Support Batterie 5V (Autodesk Fusion 360 design; units mm, degrees)
Autodesk Fusion 360 part; units mm, degrees
sketch "Sketch1" plane through (0, 0, 0) normal (0, 0, 1) x (1, 0, 0)
  circle A0 centre (0, 0) radius 11.25
  line L0 (0, 0) -> (0, -12.75) construction
  line L1 (17.5, -14.25) -> (-17.5, -14.25)
  line L2 (-17.5, -14.25) -> (-17.5, -11.25)
  line L3 (-17.5, -11.25) -> (17.5, -11.25)
  line L4 (17.5, -11.25) -> (17.5, -14.25)
  line L5 (17.5, -14.25) -> (-17.5, -11.25) construction
  line L6 (-17.5, -14.25) -> (17.5, -11.25) construction
  line L7 (11.25, -11.25) -> (13.75, -11.25)
  line L8 (13.75, -11.25) -> (13.75, 29.3)
  line L9 (11.25, 30) -> (11.25, -11.25)
  line L10 (14.45, 30) -> (14.55, 30)
  line L11 (16.75, 30) -> (16.75, 30.9)
  line L12 (15.15, 32.5) -> (12.85, 32.5)
  line L13 (11.25, 30.9) -> (11.25, 30)
  line L14 (15.25, 29.3) -> (15.25, 28)
  line L15 (15.75, 27.5) -> (16.25, 27.5)
  line L16 (16.75, 28) -> (16.75, 30)
  arc A1 (14.45, 30) -> (13.75, 29.3) centre (14.45, 29.3) ccw
  arc A2 (15.25, 29.3) -> (14.55, 30) centre (14.55, 29.3) ccw
  arc A3 (15.25, 28) -> (15.75, 27.5) centre (15.75, 28) ccw
  arc A4 (16.25, 27.5) -> (16.75, 28) centre (16.25, 28) ccw
  arc A5 (16.75, 30.9) -> (15.15, 32.5) centre (15.15, 30.9) ccw
  arc A6 (12.85, 32.5) -> (11.25, 30.9) centre (12.85, 30.9) ccw
  arc A7 (-13.75, 29.3) -> (-14.45, 30) centre (-14.45, 29.3) ccw
  line L17 (-14.45, 30) -> (-14.55, 30)
  arc A8 (-14.55, 30) -> (-15.25, 29.3) centre (-14.55, 29.3) ccw
  line L18 (-15.25, 29.3) -> (-15.25, 28)
  arc A9 (-15.75, 27.5) -> (-15.25, 28) centre (-15.75, 28) ccw
  line L19 (-15.75, 27.5) -> (-16.25, 27.5)
  arc A10 (-16.75, 28) -> (-16.25, 27.5) centre (-16.25, 28) ccw
  line L20 (-16.75, 28) -> (-16.75, 30)
  line L21 (-16.75, 30) -> (-16.75, 30.9)
  arc A11 (-15.15, 32.5) -> (-16.75, 30.9) centre (-15.15, 30.9) ccw
  line L22 (-15.15, 32.5) -> (-12.85, 32.5)
  arc A12 (-11.25, 30.9) -> (-12.85, 32.5) centre (-12.85, 30.9) ccw
  line L23 (-11.25, 30.9) -> (-11.25, 30)
  line L24 (-11.25, 30) -> (-11.25, -11.25)
  line L25 (-11.25, -11.25) -> (-13.75, -11.25)
  line L26 (-13.75, -11.25) -> (-13.75, 29.3)
  point P0 (0, -12.75)
  point P1 (16.75, 32.5)
  point P2 (16.75, 27.5)
  dimension "d1" = 22.5
  dimension "d10" = 3
  dimension "d11" = 35
  dimension "d13" = 2.5
  dimension "d14" = 30
  dimension "d16" = 5.5
  dimension "d17" = 2.5
  dimension "d19" = 2.5
  dimension "d20" = 0.7
  dimension "d21" = 0.5
  dimension "d22" = 0.5
  dimension "d23" = 1.6
  dimension "d24" = 1.5
  constraint coincident A0.centre L0.start
  constraint horizontal L1
  constraint perpendicular L1 L2
  constraint parallel L1 L3
  constraint parallel L2 L4
  constraint coincident L5 P0
  constraint coincident L6 P0
  constraint coincident P0 L0.end
  constraint tangent A0 L3
  constraint vertical L0
  constraint horizontal L7
  constraint vertical L8
  constraint vertical L9
  constraint coincident L3 L7.start
  constraint tangent A0 L9
  constraint horizontal L10
  constraint vertical L11
  constraint horizontal L12
  constraint vertical L13
  constraint vertical L14
  constraint horizontal L15
  constraint vertical L16
  constraint coincident L9.start L10
  constraint tangent L8 A1
  constraint tangent L10 A1
  constraint coincident L11.start L10
  constraint tangent L10 A2
  constraint tangent L14 A2
  constraint equal A1 A2
  constraint tangent L14 A3
  constraint tangent L15 A3
  constraint coincident P2 L15
  constraint coincident P2 L16
  constraint tangent L15 A4
  constraint tangent L16 A4
  constraint coincident P1 L11
  constraint coincident P1 L12
  constraint tangent L11 A5
  constraint tangent L12 A5
  constraint tangent L12 A6
  constraint tangent L13 A6
  constraint equal A5 A6
  constraint symmetric L0 L7.start L24.end
  constraint symmetric L0 L7.end L25.end
  constraint symmetric L0 L9.start L23.end
  constraint symmetric L0 L11.start L20.end
  constraint symmetric L0 L8.end A7.start
  constraint symmetric L0 L10.start A7.end
  constraint symmetric L0 A1 A7
  constraint symmetric L0 L10.end L17.end
  constraint symmetric L0 L14.start A8.end
  constraint symmetric L0 A2 A8
  constraint symmetric L0 L14.end L18.end
  constraint symmetric L0 L15.start A9.start
  constraint symmetric L0 A3 A9
  constraint symmetric L0 L15.end L19.end
  constraint symmetric L0 L16.start A10.start
  constraint symmetric L0 A4 A10
  constraint symmetric L0 L11.end L21.end
  constraint symmetric L0 L12.start A11.start
  constraint symmetric L0 A5 A11
  constraint symmetric L0 L12.end L22.end
  constraint symmetric L0 L13.start A12.start
  constraint symmetric L0 A6 A12
  measures "d1" diameter of A0
  measures "d10" distance of L1.end L2.end
  measures "d11" distance of L1.start L1.end
  measures "d13" distance of L7.start L7.end
  measures "d14" vertical distance of A0.centre L9.start
  measures "d16" distance of L9.start L11.start
  measures "d17" distance of L11.start P1
  measures "d19" distance of L11.start P2
  measures "d20" radius of A1
  measures "d21" radius of A3
  measures "d22" radius of A4
  measures "d23" radius of A5
  measures "d24" distance of L14 L16
extrude "Extrude1" add sketch "Sketch1" along normal blind 30 contours A0 L3 L9 | L3 L7 L8 L9 L10 L11 L12 L13 L14 L15 L16 A1 A2 A3 A4 A5 A6 | L3 A7 L17 A8 L18 A9 L19 A10 L20 L21 A11 L22 A12 L23 L24 L25 L26 | A0 L3 L24 | L1 L2 L3 L4 L7 L25
fillet "Fillet1" radius 7.5 2 edges at (-13.75, -11.25, 15) (13.75, -11.25, 15)
sketch "Sketch2" plane through (0, -14.25, 0) normal (0, -1, 0) x (1, 0, 0)
  line L0 (-17.5, 0) -> (17.5, 0)
  line L1 (17.5, 0) -> (17.5, 30)
  line L2 (17.5, 30) -> (-17.5, 30)
  line L3 (-17.5, 30) -> (-17.5, 0)
  line L4 (0, 0) -> (0, 18) construction
  line L5 (-5, 18) -> (5, 18)
  circle A0 centre (-5, 18) radius 1.5
  circle A1 centre (5, 18) radius 1.5
  dimension "d29" = 18
  dimension "d30" = 10
  dimension "d31" = 3
  dimension "d32" = 3
  constraint coincident L4.start origin
  constraint perpendicular L0 L4
  constraint perpendicular L4 L5
  constraint coincident L4.end L5
  constraint midpoint L4.end L5
  constraint coincident L5.start A0.centre
  constraint coincident L5.end A1.centre
  measures "d29" distance of L4.start L4.end
  measures "d30" distance of L5.start L5.end
  measures "d31" diameter of A0
  measures "d32" diameter of A1
extrude "Extrude2" cut sketch "Sketch2" against normal through all contours A0 | A1
ref_plane "WorkPlane1" through (0, -11.25, 15) normal (0, -1, 0) x (1, 0, 0)
sketch "Sketch4" plane through (0, -11.25, 15) normal (0, -1, 0) x (1, 0, 0)
  circle A0 centre (-5, 3) radius 1.5
  circle A1 centre (5, 3) radius 1.5
  circle A2 centre (-5, 3) radius 3
  circle A3 centre (5, 3) radius 3
  dimension "d38" = 6
  dimension "d39" = 6
  constraint concentric A0 A2
  constraint concentric A1 A3
  measures "d38" diameter of A2
  measures "d39" diameter of A3
extrude "Extrude4" cut sketch "Sketch4" against normal blind 14
sketch "Sketch5" plane through (0, 0, 0) normal (0, 0, -1) x (1, 0, 0)
  arc A0 (17.5, 11.25) -> (13.75, 4.7548) centre (21.25, 4.7548) ccw
  line L0 (17.5, 11.25) -> (17.5, 14.25)
  line L1 (17.5, 14.25) -> (-17.5, 14.25)
  line L2 (-17.5, 14.25) -> (-17.5, 11.25)
  arc A1 (-13.75, 4.7548) -> (-17.5, 11.25) centre (-21.25, 4.7548) ccw
  line L3 (-13.75, 4.7548) -> (-13.75, -29.3)
  arc A2 (-14.45, -30) -> (-13.75, -29.3) centre (-14.45, -29.3) ccw
  line L4 (-14.45, -30) -> (-14.55, -30)
  arc A3 (-15.25, -29.3) -> (-14.55, -30) centre (-14.55, -29.3) ccw
  line L5 (-15.25, -29.3) -> (-15.25, -28)
  arc A4 (-15.25, -28) -> (-15.75, -27.5) centre (-15.75, -28) ccw
  line L6 (-15.75, -27.5) -> (-16.25, -27.5)
  arc A5 (-16.25, -27.5) -> (-16.75, -28) centre (-16.25, -28) ccw
  line L7 (-16.75, -28) -> (-16.75, -30.9)
  arc A6 (-16.75, -30.9) -> (-15.15, -32.5) centre (-15.15, -30.9) ccw
  line L8 (-15.15, -32.5) -> (-12.85, -32.5)
  arc A7 (-12.85, -32.5) -> (-11.25, -30.9) centre (-12.85, -30.9) ccw
  line L9 (-11.25, -30.9) -> (-11.25, 0)
  arc A8 (11.25, 0) -> (-11.25, 0) centre (0, 0) ccw
  line L10 (11.25, 0) -> (11.25, -30.9)
  arc A9 (11.25, -30.9) -> (12.85, -32.5) centre (12.85, -30.9) ccw
  line L11 (12.85, -32.5) -> (15.15, -32.5)
  arc A10 (15.15, -32.5) -> (16.75, -30.9) centre (15.15, -30.9) ccw
  line L12 (16.75, -30.9) -> (16.75, -28)
  arc A11 (16.75, -28) -> (16.25, -27.5) centre (16.25, -28) ccw
  line L13 (16.25, -27.5) -> (15.75, -27.5)
  arc A12 (15.75, -27.5) -> (15.25, -28) centre (15.75, -28) ccw
  line L14 (15.25, -28) -> (15.25, -29.3)
  arc A13 (14.55, -30) -> (15.25, -29.3) centre (14.55, -29.3) ccw
  line L15 (14.55, -30) -> (14.45, -30)
  arc A14 (13.75, -29.3) -> (14.45, -30) centre (14.45, -29.3) ccw
  line L16 (13.75, -29.3) -> (13.75, 4.7548)
  line L17 (-11.25, 0) -> (11.25, 0)
  constraint coincident L9.end A8.end
  constraint coincident A8.start L10.start
extrude "Extrude5" add sketch "Sketch5" along normal blind 3
sketch "Sketch6" plane through (0, 32.5, 0) normal (0, 1, 0) x (-1, 0, 0)
  line L0 (15.15, -3) -> (15.15, 30)
  line L1 (15.15, 30) -> (12.85, 30)
  line L2 (12.85, 30) -> (12.85, -3)
  line L3 (12.85, -3) -> (15.15, -3)
  line L4 (-12.85, -3) -> (-12.85, 30)
  line L5 (-12.85, 30) -> (-15.15, 30)
  line L6 (-15.15, 30) -> (-15.15, -3)
  line L7 (-15.15, -3) -> (-12.85, -3)
  line L8 (-15.15, 18.5) -> (-22.1698, 18.5)
  line L9 (-22.1698, 18.5) -> (-22.1698, 8.5)
  line L10 (-22.1698, 8.5) -> (-15.15, 8.5)
  line L11 (-15.15, 8.5) -> (-15.15, 18.5)
  line L12 (15.15, 18.5) -> (21.4643, 18.5)
  line L13 (21.4643, 18.5) -> (21.4643, 8.5)
  line L14 (21.4643, 8.5) -> (15.15, 8.5)
  line L15 (15.15, 8.5) -> (15.15, 18.5)
  line L16 (15.15, 18.5) -> (13.85, 18.5)
  line L17 (13.85, 18.5) -> (13.85, 8.5)
  line L18 (13.85, 8.5) -> (15.15, 8.5)
  line L19 (15.15, 8.5) -> (15.15, 18.5)
  line L20 (-15.15, 18.5) -> (-13.85, 18.5)
  line L21 (-13.85, 18.5) -> (-13.85, 8.5)
  line L22 (-13.85, 8.5) -> (-15.15, 8.5)
  line L23 (-15.15, 8.5) -> (-15.15, 18.5)
  dimension "d44" = 10
  dimension "d45" = 10
  dimension "d48" = 1.3
  dimension "d49" = 1.3
  constraint horizontal L8
  constraint vertical L9
  constraint horizontal L10
  constraint vertical L11
  constraint coincident L6 L8.start
  constraint horizontal L12
  constraint vertical L13
  constraint horizontal L14
  constraint vertical L15
  constraint coincident L0 L12.start
  constraint midpoint L6 L11
  constraint midpoint L0 L15
  constraint horizontal L16
  constraint vertical L17
  constraint horizontal L18
  constraint vertical L19
  constraint coincident L14.end L15.start
  constraint horizontal L20
  constraint vertical L21
  constraint horizontal L22
  constraint vertical L23
  constraint coincident L10.end L11.start
  measures "d44" distance of L8.start L10.end
  measures "d45" distance of L12.start L14.end
  measures "d48" distance of L12.start L16.end
  measures "d49" distance of L8.start L20.end
extrude "Extrude6" cut sketch "Sketch6" against normal blind 9 contours L0 L15 L16 L17 L18 L19 | L0 L12 L13 L14 L15 L19 | L6 L8 L9 L10 L11 L23 | L6 L11 L20 L21 L22 L23
named bodies: "Support_Bat5V"
